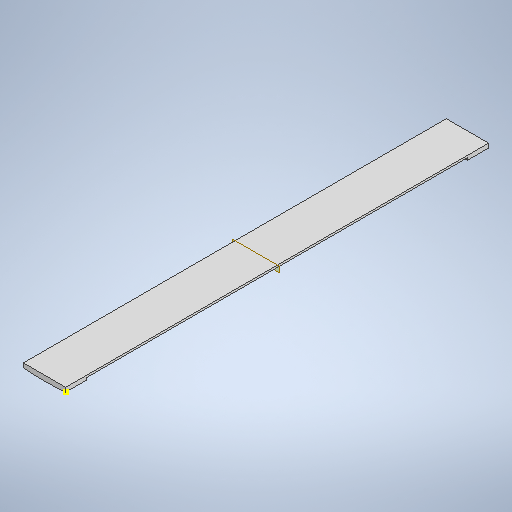
# Autodesk Inventor part: Lock
Saved by Autodesk Inventor 2025 (Build 290162010, 162A)
## iProperties
Created: 2024-06-06
Part Number: Lock
Material: Generic
Document SubType Name: Modeling
Designer: vncnt
Density: 1 g/cm^3
Appearance: Default
Author: vncnt
Autodesk Inventor part; units mm, degrees
ref_plane "YZ Plane" through (0, 0, 0) normal (1, 0, 0) x (0, 1, 0)
ref_plane "XZ Plane" through (0, 0, 0) normal (0, 1, 0) x (-1, 0, 0)
ref_plane "XY Plane" through (0, 0, 0) normal (0, 0, 1) x (1, 0, 0)
sketch "Sketch1" plane through (0, 0, 0) normal (0, 1, 0) x (-1, 0, 0)
  line L0 (0, 0) -> (-2.54, 0)
  line L1 (-2.54, 0) -> (-2.54, -25.4)
  line L2 (-2.54, -25.4) -> (0, -25.4)
  line L3 (0, -25.4) -> (0, 0)
  dimension "d0" = 2.54
  dimension "d1" = 25.4
  constraints: 8 end point, 2 parallel, 1 horizontal, 1 perpendicular
  measures "d0" distance of L2.end L1.end
  measures "d1" distance of L1.end L0.end
extrude "Extrusion1" add sketch "Sketch1" along normal blind 0.254
sketch "Sketch2" plane through (0, 0, 0) normal (0, 0, 1) x (1, 0, 0)
  arc A0 (0, 0) -> (2.54, 0) centre (1.27, 14.1672) ccw
  line L0 (0, 0) -> (2.54, 0)
  dimension "d5" = 14.224
  constraints: 2 end point, 2 point on circle, 1 centre point, 1 horizontal
  measures "d5" radius of A0
extrude "Extrusion2" add sketch "Sketch2" against normal blind 1.27
sketch "Sketch3" plane through (2.54, 0.254, 0) normal (1, 0, 0) x (0, 0, -1)
  point P0 (0, -0.254)
ref_plane "Work Plane1" through (0, 0.254, -12.7) normal (0, 0, 1) x (1, 0, 0)
mirror "Mirror1" about plane through (0, 0.254, -12.7) normal (0, 0, 1) of "Extrusion2"
sketch "Sketch4" plane through (2.54, 0.254, 0) normal (1, 0, 0) x (0, 0, -1)
  line L0 (24.1358, -0.254) -> (1.27, -0.254)
  line L1 (1.27, -0.254) -> (1.27, -0.1226)
  line L2 (1.27, -0.1226) -> (24.1358, -0.1226)
  line L3 (24.1358, -0.1226) -> (24.1358, -0.254)
  point P0 (0, -0.254)
  constraints: 8 end point, 2 parallel, 1 horizontal, 1 perpendicular
extrude "Extrusion3" cut sketch "Sketch4" against normal blind 25.4
ref_plane "Work Plane2" through (0, 0.254, -12.7) normal (0, 0, 1) x (1, 0, 0)
body "Solid1"
